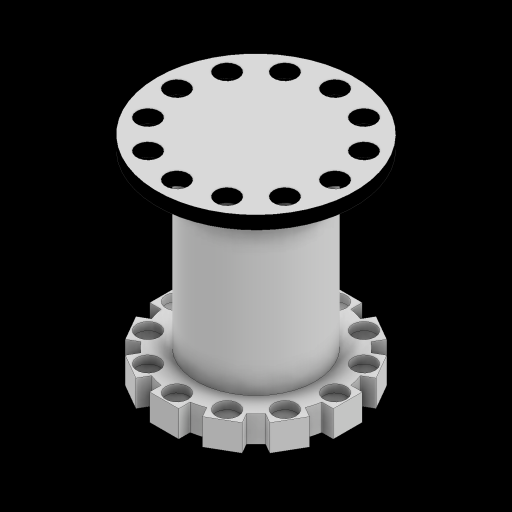
# Autodesk Inventor part: SC-1-02-Test Tube Rack
Saved by Autodesk Inventor 2023 (Build 270158000, 158)
## iProperties
Created: 2022-10-22
Part Number: SC-1-02-Test Tube Rack
Material: Generic
Document SubType Name: Modeling
Designer: annah
Density: 1 g/cm^3
Appearance: Default
Author: annah
Autodesk Inventor part; units mm, degrees
ref_plane "YZ Plane" through (0, 0, 0) normal (1, 0, 0) x (0, 1, 0)
ref_plane "XZ Plane" through (0, 0, 0) normal (0, 1, 0) x (-1, 0, 0)
ref_plane "XY Plane" through (0, 0, 0) normal (0, 0, 1) x (1, 0, 0)
sketch "Sketch1" plane through (0, 0, 0) normal (0, 1, 0) x (-1, 0, 0)
  circle A0 centre (0, 0) radius 75
  circle A1 centre (0, 0) radius 60
  circle A2 centre (0, 60) radius 8.5
  circle A3 centre (-30, 51.9615) radius 8.5
  circle A4 centre (-51.9615, 30) radius 8.5
  circle A5 centre (-60, 0) radius 8.5
  circle A6 centre (-51.9615, -30) radius 8.5
  circle A7 centre (-30, -51.9615) radius 8.5
  circle A8 centre (0, -60) radius 8.5
  circle A9 centre (30, -51.9615) radius 8.5
  circle A10 centre (51.9615, -30) radius 8.5
  circle A11 centre (60, 0) radius 8.5
  circle A12 centre (51.9615, 30) radius 8.5
  circle A13 centre (30, 51.9615) radius 8.5
  dimension "d1" = 120
  dimension "d0" = 150
  dimension "d2" = 17
  dimension "d5" = 360
  constraints: 13 centre point, 2 coincident, 1 vertical alignment, 27 other
  measures "d0" diameter of A0
  measures "d2" diameter of A2
extrude "Extrusion1" add sketch "Sketch1" along normal blind 10 contours A0 | A11 A1 A10 A9 A8 A7 A6 A5 A4 A3 A2 A13 A12
sketch "Sketch2" plane through (0, 0, 0) normal (0, -1, 0) x (1, 0, 0)
  circle A0 centre (0, 0) radius 45
  dimension "d9" = 90
  constraints: 1 centre point, 1 coincident
  measures "d9" diameter of A0
extrude "Extrusion2" add sketch "Sketch2" along normal blind 130
sketch "Sketch3" plane through (0, -130, 0) normal (0, -1, 0) x (1, 0, 0)
  circle A0 centre (0, 0) radius 5
  line L0 (-11.0031, 74.0969) -> (11.0031, 74.0969)
  line L1 (11.0031, 74.0969) -> (11.0031, 56.269)
  line L2 (11.0031, 56.269) -> (-11.0031, 56.269)
  line L3 (-11.0031, 56.269) -> (-11.0031, 74.0969)
  line L4 (11.0031, 74.0969) -> (0, 65.183) construction
  line L5 (-27.5195, 69.6713) -> (-18.6056, 54.232)
  line L6 (-18.6056, 54.232) -> (-37.6635, 43.2289)
  line L7 (-37.6635, 43.2289) -> (-46.5774, 58.6682)
  line L8 (-46.5774, 58.6682) -> (-27.5195, 69.6713)
  line L9 (-58.6682, 46.5774) -> (-43.2289, 37.6635)
  line L10 (-43.2289, 37.6635) -> (-54.232, 18.6056)
  line L11 (-54.232, 18.6056) -> (-69.6713, 27.5195)
  line L12 (-69.6713, 27.5195) -> (-58.6682, 46.5774)
  line L13 (-74.0969, 11.0031) -> (-56.269, 11.0031)
  line L14 (-56.269, 11.0031) -> (-56.269, -11.0031)
  line L15 (-56.269, -11.0031) -> (-74.0969, -11.0031)
  line L16 (-74.0969, -11.0031) -> (-74.0969, 11.0031)
  line L17 (-69.6713, -27.5195) -> (-54.232, -18.6056)
  line L18 (-54.232, -18.6056) -> (-43.2289, -37.6635)
  line L19 (-43.2289, -37.6635) -> (-58.6682, -46.5774)
  line L20 (-58.6682, -46.5774) -> (-69.6713, -27.5195)
  line L21 (-46.5774, -58.6682) -> (-37.6635, -43.2289)
  line L22 (-37.6635, -43.2289) -> (-18.6056, -54.232)
  line L23 (-18.6056, -54.232) -> (-27.5195, -69.6713)
  line L24 (-27.5195, -69.6713) -> (-46.5774, -58.6682)
  line L25 (-11.0031, -74.0969) -> (-11.0031, -56.269)
  line L26 (-11.0031, -56.269) -> (11.0031, -56.269)
  line L27 (11.0031, -56.269) -> (11.0031, -74.0969)
  line L28 (11.0031, -74.0969) -> (-11.0031, -74.0969)
  line L29 (27.5195, -69.6713) -> (18.6056, -54.232)
  line L30 (18.6056, -54.232) -> (37.6635, -43.2289)
  line L31 (37.6635, -43.2289) -> (46.5774, -58.6682)
  line L32 (46.5774, -58.6682) -> (27.5195, -69.6713)
  line L33 (58.6682, -46.5774) -> (43.2289, -37.6635)
  line L34 (43.2289, -37.6635) -> (54.232, -18.6056)
  line L35 (54.232, -18.6056) -> (69.6713, -27.5195)
  line L36 (69.6713, -27.5195) -> (58.6682, -46.5774)
  line L37 (74.0969, -11.0031) -> (56.269, -11.0031)
  line L38 (56.269, -11.0031) -> (56.269, 11.0031)
  line L39 (56.269, 11.0031) -> (74.0969, 11.0031)
  line L40 (74.0969, 11.0031) -> (74.0969, -11.0031)
  line L41 (69.6713, 27.5195) -> (54.232, 18.6056)
  line L42 (54.232, 18.6056) -> (43.2289, 37.6635)
  line L43 (43.2289, 37.6635) -> (58.6682, 46.5774)
  line L44 (58.6682, 46.5774) -> (69.6713, 27.5195)
  line L45 (46.5774, 58.6682) -> (37.6635, 43.2289)
  line L46 (37.6635, 43.2289) -> (18.6056, 54.232)
  line L47 (18.6056, 54.232) -> (27.5195, 69.6713)
  line L48 (27.5195, 69.6713) -> (46.5774, 58.6682)
  arc A1 (-11.0031, 60.9667) -> (-20.9544, 58.3003) centre (0, 0) ccw
  arc A2 (20.9544, 58.3003) -> (11.0031, 60.9667) centre (0, 0) ccw
  arc A3 (47.2972, 40.0123) -> (40.0123, 47.2972) centre (0, 0) ccw
  arc A4 (-40.0123, 47.2972) -> (-47.2972, 40.0123) centre (0, 0) ccw
  arc A5 (-58.3003, 20.9544) -> (-60.9667, 11.0031) centre (0, 0) ccw
  arc A6 (-60.9667, -11.0031) -> (-58.3003, -20.9544) centre (0, 0) ccw
  arc A7 (-47.2972, -40.0123) -> (-40.0123, -47.2972) centre (0, 0) ccw
  arc A8 (-20.9544, -58.3003) -> (-11.0031, -60.9667) centre (0, 0) ccw
  arc A9 (11.0031, -60.9667) -> (20.9544, -58.3003) centre (0, 0) ccw
  arc A10 (40.0123, -47.2972) -> (47.2972, -40.0123) centre (0, 0) ccw
  arc A11 (58.3003, -20.9544) -> (60.9667, -11.0031) centre (0, 0) ccw
  arc A12 (60.9667, 11.0031) -> (58.3003, 20.9544) centre (0, 0) ccw
  circle A13 centre (0, 0) radius 59.8407
  line L49 (-69.6713, -11.0031) -> (-49.8173, -11.0031)
  line L50 (-49.8173, -11.0031) -> (-49.8173, 11.0031)
  line L51 (-49.8173, 11.0031) -> (-69.6713, 11.0031)
  line L52 (-69.6713, 11.0031) -> (-69.6713, -11.0031)
  line L53 (-74.0969, 11.0031) -> (-56.269, 11.0031)
  line L54 (-65.8387, -25.3067) -> (-54.8356, -44.3646)
  line L55 (-48.6446, -15.3797) -> (-65.8387, -25.3067)
  line L56 (-37.6415, -34.4376) -> (-48.6446, -15.3797)
  line L57 (-54.8356, -44.3646) -> (-37.6415, -34.4376)
  line L58 (-69.6713, -27.5195) -> (-54.232, -18.6056)
  line L59 (-44.3646, -54.8356) -> (-25.3067, -65.8387)
  line L60 (-34.4376, -37.6415) -> (-44.3646, -54.8356)
  line L61 (-15.3797, -48.6446) -> (-34.4376, -37.6415)
  line L62 (-25.3067, -65.8387) -> (-15.3797, -48.6446)
  line L63 (-46.5774, -58.6682) -> (-37.6635, -43.2289)
  line L64 (-11.0031, -69.6713) -> (11.0031, -69.6713)
  line L65 (-11.0031, -49.8173) -> (-11.0031, -69.6713)
  line L66 (11.0031, -49.8173) -> (-11.0031, -49.8173)
  line L67 (11.0031, -69.6713) -> (11.0031, -49.8173)
  line L68 (-11.0031, -74.0969) -> (-11.0031, -56.269)
  line L69 (25.3067, -65.8387) -> (44.3646, -54.8356)
  line L70 (15.3797, -48.6446) -> (25.3067, -65.8387)
  line L71 (34.4376, -37.6415) -> (15.3797, -48.6446)
  line L72 (44.3646, -54.8356) -> (34.4376, -37.6415)
  line L73 (27.5195, -69.6713) -> (18.6056, -54.232)
  line L74 (54.8356, -44.3646) -> (65.8387, -25.3067)
  line L75 (37.6415, -34.4376) -> (54.8356, -44.3646)
  line L76 (48.6446, -15.3797) -> (37.6415, -34.4376)
  line L77 (65.8387, -25.3067) -> (48.6446, -15.3797)
  line L78 (58.6682, -46.5774) -> (43.2289, -37.6635)
  line L79 (69.6713, -11.0031) -> (69.6713, 11.0031)
  line L80 (49.8173, -11.0031) -> (69.6713, -11.0031)
  line L81 (49.8173, 11.0031) -> (49.8173, -11.0031)
  line L82 (69.6713, 11.0031) -> (49.8173, 11.0031)
  line L83 (74.0969, -11.0031) -> (56.269, -11.0031)
  line L84 (65.8387, 25.3067) -> (54.8356, 44.3646)
  line L85 (48.6446, 15.3797) -> (65.8387, 25.3067)
  line L86 (37.6415, 34.4376) -> (48.6446, 15.3797)
  line L87 (54.8356, 44.3646) -> (37.6415, 34.4376)
  line L88 (69.6713, 27.5195) -> (54.232, 18.6056)
  line L89 (44.3646, 54.8356) -> (25.3067, 65.8387)
  line L90 (34.4376, 37.6415) -> (44.3646, 54.8356)
  line L91 (15.3797, 48.6446) -> (34.4376, 37.6415)
  line L92 (25.3067, 65.8387) -> (15.3797, 48.6446)
  line L93 (46.5774, 58.6682) -> (37.6635, 43.2289)
  line L94 (11.0031, 69.6713) -> (-11.0031, 69.6713)
  line L95 (11.0031, 49.8173) -> (11.0031, 69.6713)
  line L96 (-11.0031, 49.8173) -> (11.0031, 49.8173)
  line L97 (-11.0031, 69.6713) -> (-11.0031, 49.8173)
  line L98 (11.0031, 74.0969) -> (11.0031, 56.269)
  line L99 (-25.3067, 65.8387) -> (-44.3646, 54.8356)
  line L100 (-15.3797, 48.6446) -> (-25.3067, 65.8387)
  line L101 (-34.4376, 37.6415) -> (-15.3797, 48.6446)
  line L102 (-44.3646, 54.8356) -> (-34.4376, 37.6415)
  line L103 (-27.5195, 69.6713) -> (-18.6056, 54.232)
  line L104 (-54.8356, 44.3646) -> (-65.8387, 25.3067)
  line L105 (-37.6415, 34.4376) -> (-54.8356, 44.3646)
  line L106 (-48.6446, 15.3797) -> (-37.6415, 34.4376)
  line L107 (-65.8387, 25.3067) -> (-48.6446, 15.3797)
  point P0 (-58.3003, -20.9544)
  point P1 (-11.0031, -60.9667)
  point P2 (20.9544, -58.3003)
  point P3 (47.2972, -40.0123)
  point P4 (60.9667, -11.0031)
  point P5 (58.3003, 20.9544)
  point P6 (40.0123, 47.2972)
  point P7 (11.0031, 60.9667)
  point P8 (-20.9544, 58.3003)
  dimension "d68" = 360
  dimension "d105" = 360
  constraints: 216 end point, 36 point on line, 24 point on circle, 14 centre point, 4 coincident, 4 parallel, 2 horizontal, 2 perpendicular, 242 other
extrude "Extrusion9" add sketch "Sketch3" along normal blind 20 contours L94 L1 A13 L3 | L3 A13 L5 A1 | A2 L47 A13 L1 | A13 L1 L2 L3 | L3 L97 L96 L95 L1 A13 L47 L92 L91 L90 L45 L43 L87 L86 L85 L41 L39 L82 L81 L80 L37 L35 L77 L76 L75 L33 L31 L72 L71 L70 L29 L27 L67 L66 L65 L25 L23 L62 L61 L60 L21 L19 L57 L56 L55 L17 L15 L49 L50 L51 L13 L11 L107 L106 L105 L9 L7 L102 L101 L100 L5 | L5 A13 L7 L99 | L47 L89 L45 A13 | L2 L95 L96 L97 | L5 L6 L7 A13 | A13 L45 L46 L47 | L100 L101 L102 L6 | A13 L9 A4 L7 | L46 L90 L91 L92 | L45 A3 L43 A13 | A13 L11 L104 L9 | L9 L10 L11 A13 | A13 L41 L42 L43 | L43 L84 L41 A13 | L105 L106 L107 L10 | A13 L13 A5 L11 | L42 L85 L86 L87 | L41 A12 L39 A13 | A13 L15 L52 L13 | L13 L14 L15 A13 | A13 L37 L38 L39 | L39 L79 L37 A13 | L51 L50 L49 L14 | A13 L17 A6 L15 | L38 L80 L81 L82 | A13 L19 L54 L17 | L17 L18 L19 A13 | L37 A11 L35 A13 | L55 L56 L57 L18 | A13 L21 A7 L19 | A13 L33 L34 L35 | L35 L74 L33 A13 | A13 L23 L59 L21 | L21 L22 L23 A13 | L34 L75 L76 L77 | L33 A10 L31 A13 | L60 L61 L62 L22 | A13 L25 A8 L23 | A13 L29 L30 L31 | L31 L69 L29 A13 | A13 L27 L64 L25 | L25 L26 L27 A13 | L30 L70 L71 L72 | L29 A9 L27 A13 | L65 L66 L67 L26
sketch "Sketch7" plane through (0, -130, 0) normal (0, 1, 0) x (1, 0, 0)
  circle A0 centre (0, 0) radius 5 projected
  circle A1 centre (0, 0) radius 60
  circle A2 centre (-60, 0) radius 8.5
  circle A3 centre (-51.9615, -30) radius 8.5
  circle A4 centre (-30, -51.9615) radius 8.5
  circle A5 centre (0, -60) radius 8.5
  circle A6 centre (30, -51.9615) radius 8.5
  circle A7 centre (51.9615, -30) radius 8.5
  circle A8 centre (60, 0) radius 8.5
  circle A9 centre (51.9615, 30) radius 8.5
  circle A10 centre (30, 51.9615) radius 8.5
  circle A11 centre (0, 60) radius 8.5
  circle A12 centre (-30, 51.9615) radius 8.5
  circle A13 centre (-51.9615, 30) radius 8.5
  dimension "d71" = 120
  dimension "d72" = 17
  dimension "d75" = 360
  constraints: 12 centre point, 1 coincident, 1 horizontal alignment, 27 other
  measures "d72" diameter of A2
extrude "Extrusion10" cut sketch "Sketch7" against normal blind 10 contours A1 A8 | A1 A8 | A9 A1 | A1 A9 | A7 A1 | A1 A7 | A10 A1 | A1 A10 | A6 A1 | A1 A6 | A11 A1 | A1 A11 | A5 A1 | A1 A5 | A12 A1 | A1 A12 | A4 A1 | A1 A4 | A13 A1 | A1 A13 | A3 A1 | A1 A3 | A2 A1 | A1 A2
fillet "Fillet1" radius 4 12 edges at (-68.5, -140, 0) (-60.4615, -140, -30) (-60.4615, -140, 30) (-38.5, -140, 51.9615) (-8.5, -140, 60) (21.5, -140, 51.9615) (43.4615, -140, 30) (51.5, -140, 0) (-38.5, -140, -51.9615) (-8.5, -140, -60) (21.5, -140, -51.9615) (43.4615, -140, -30)
sketch "Sketch8" plane through (0, -150, 0) normal (0, -1, 0) x (1, 0, 0)
  circle A0 centre (0, 0) radius 62.2015
  line L0 (11.5029, -60.4669) -> (-11.5031, -60.4669)
  line L1 (-11.5031, -60.4669) -> (-11.5031, -74.5969)
  line L2 (-11.0031, -60.9667) -> (-11.0031, -69.6713) projected
  line L3 (11.0031, -69.6713) -> (11.0031, -60.9667) projected
  line L4 (-11.5031, -74.5969) -> (11.5029, -74.5969)
  line L5 (11.5029, -60.4669) -> (11.5029, -74.5969)
  line L6 (-11.0031, -74.0969) -> (11.0031, -74.0969) projected
  line L7 (40.1952, -46.6144) -> (20.2715, -58.1174)
  line L8 (40.1952, -46.6144) -> (47.2602, -58.8513)
  line L9 (27.3365, -70.3543) -> (47.2602, -58.8513)
  line L10 (20.2715, -58.1174) -> (27.3365, -70.3543)
  line L11 (58.1173, -20.2716) -> (46.6143, -40.1954)
  line L12 (58.1173, -20.2716) -> (70.3542, -27.3366)
  line L13 (58.8512, -47.2604) -> (70.3542, -27.3366)
  line L14 (46.6143, -40.1954) -> (58.8512, -47.2604)
  line L15 (60.4669, 11.5029) -> (60.4669, -11.5031)
  line L16 (60.4669, 11.5029) -> (74.5969, 11.5029)
  line L17 (74.5969, -11.5031) -> (74.5969, 11.5029)
  line L18 (60.4669, -11.5031) -> (74.5969, -11.5031)
  line L19 (46.6144, 40.1952) -> (58.1174, 20.2715)
  line L20 (46.6144, 40.1952) -> (58.8513, 47.2602)
  line L21 (70.3543, 27.3365) -> (58.8513, 47.2602)
  line L22 (58.1174, 20.2715) -> (70.3543, 27.3365)
  line L23 (20.2716, 58.1173) -> (40.1954, 46.6143)
  line L24 (20.2716, 58.1173) -> (27.3366, 70.3542)
  line L25 (47.2604, 58.8512) -> (27.3366, 70.3542)
  line L26 (40.1954, 46.6143) -> (47.2604, 58.8512)
  line L27 (-11.5029, 60.4669) -> (11.5031, 60.4669)
  line L28 (-11.5029, 60.4669) -> (-11.5029, 74.5969)
  line L29 (11.5031, 74.5969) -> (-11.5029, 74.5969)
  line L30 (11.5031, 60.4669) -> (11.5031, 74.5969)
  line L31 (-40.1952, 46.6144) -> (-20.2715, 58.1174)
  line L32 (-40.1952, 46.6144) -> (-47.2602, 58.8513)
  line L33 (-27.3365, 70.3543) -> (-47.2602, 58.8513)
  line L34 (-20.2715, 58.1174) -> (-27.3365, 70.3543)
  line L35 (-58.1173, 20.2716) -> (-46.6143, 40.1954)
  line L36 (-58.1173, 20.2716) -> (-70.3542, 27.3366)
  line L37 (-58.8512, 47.2604) -> (-70.3542, 27.3366)
  line L38 (-46.6143, 40.1954) -> (-58.8512, 47.2604)
  line L39 (-60.4669, -11.5029) -> (-60.4669, 11.5031)
  line L40 (-60.4669, -11.5029) -> (-74.5969, -11.5029)
  line L41 (-74.5969, 11.5031) -> (-74.5969, -11.5029)
  line L42 (-60.4669, 11.5031) -> (-74.5969, 11.5031)
  line L43 (-46.6144, -40.1952) -> (-58.1174, -20.2715)
  line L44 (-46.6144, -40.1952) -> (-58.8513, -47.2602)
  line L45 (-70.3543, -27.3365) -> (-58.8513, -47.2602)
  line L46 (-58.1174, -20.2715) -> (-70.3543, -27.3365)
  line L47 (-20.2716, -58.1173) -> (-40.1954, -46.6143)
  line L48 (-20.2716, -58.1173) -> (-27.3366, -70.3542)
  line L49 (-47.2604, -58.8512) -> (-27.3366, -70.3542)
  line L50 (-40.1954, -46.6143) -> (-47.2604, -58.8512)
  dimension "d92" = 124.403
  dimension "d93" = 23.006
  dimension "d94" = 14.13
  dimension "d95" = 0.5
  dimension "d97" = 14.13
  dimension "d98" = 0.5
  dimension "d101" = 360
  constraints: 96 end point, 1 centre point, 1 coincident, 1 horizontal, 1 vertical, 97 other
  measures "d92" diameter of A0
  measures "d93" distance of L0.start L0.end
  measures "d94" distance of L0.end L1.end
  measures "d95" distance between parallel lines of L2 L1
  measures "d97" distance of L0.start L4.end
  measures "d98" distance between parallel lines of L6 L4
equation "\"d94\" = d97"
body "Solid1"
